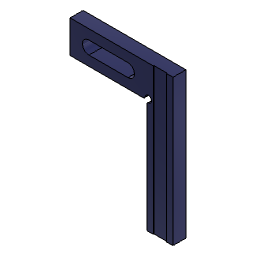
Square_Class (Autodesk Fusion 360 archive; units mm, degrees)
design "Square_Bottom"
Autodesk Fusion 360 part; units mm, degrees
sketch "Sketch1" plane through (0, 0, 0) normal (0, 1, 0) x (1, 0, 0)
  line L0 (0, 0) -> (20, 0)
  line L1 (20, 0) -> (20, -112)
  line L2 (20, -112) -> (-59, -112)
  line L3 (-59, -112) -> (-59, -87)
  line L4 (-59, -87) -> (-2.4388, -87)
  line L5 (0, 0) -> (0, -84.5612)
  line L6 (0, -87) -> (1.0607, -88.0607) construction
  line L7 (0, -87) -> (2, -87) construction
  arc A0 (-1.439, -88.0173) -> (1.0173, -85.561) centre (1.0607, -88.0607) ccw
  arc A1 (0, -84.5612) -> (1.0173, -85.561) centre (1, -84.5612) ccw
  arc A2 (-1.439, -88.0173) -> (-2.4388, -87) centre (-2.4388, -88) ccw
  line L8 (-59, -99.5) -> (-49.5, -99.5) construction
  line L9 (-27.9553, -112) -> (-27.9553, -104.5) construction
  line L10 (-27.9553, -87) -> (-27.9553, -94.5) construction
  line L11 (-14.5, -94.5) -> (-44.5, -94.5)
  line L12 (-44.5, -104.5) -> (-14.5, -104.5)
  arc A3 (-14.5, -104.5) -> (-14.5, -94.5) centre (-14.5, -99.5) ccw
  arc A4 (-44.5, -94.5) -> (-44.5, -104.5) centre (-44.5, -99.5) ccw
  point P0 (0, -85.7968)
  dimension "d1" = 20
  dimension "d2" = 112
  dimension "d3" = 79
  dimension "d5" = 59
  dimension "d8" = 45
  dimension "d9" = 1.5
  dimension "d10" = 5
  dimension "d11" = 25
  dimension "d12" = 85.7968
  dimension "d13" = 1
  dimension "d14" = 9.5
  dimension "d15" = 7.5
  dimension "d16" = 7.5
  dimension "d17" = 10
  dimension "d18" = 30
  dimension "d19" = 10
  constraint coincident L0.start L5.start
  constraint horizontal L0
  constraint perpendicular L0 L1
  constraint perpendicular L1 L2
  constraint perpendicular L2 L3
  constraint perpendicular L3 L4
  constraint horizontal L7
  constraint coincident L6.end A0.centre
  constraint coincident L5 P0
  constraint coincident P0 A0
  constraint tangent L5 A1
  constraint tangent A0 A1
  constraint tangent L4 A2
  constraint tangent A0 A2
  constraint equal A1 A2
  constraint midpoint L3 L8.start
  constraint perpendicular L3 L8
  constraint coincident L2 L9.start
  constraint perpendicular L2 L9
  constraint coincident L4 L10.start
  constraint perpendicular L4 L10
  constraint coincident L8.end A4
  constraint tangent L11 A4
  constraint perpendicular L10 L11
  constraint tangent L12 A3
  constraint perpendicular L9 L12
  measures "d1" distance of L0.start L0.end
  measures "d2" distance of L0.end L1.end
  measures "d3" distance of L1.end L2.end
  measures "d5" distance of L3.end L6.start
  measures "d8" angle of L6 L7
  measures "d9" distance of L6.start L6.end
  measures "d10" diameter of A0
  measures "d11" distance of L2 L4
  measures "d12" distance of L0.start P0
  measures "d13" radius of A1
  measures "d14" distance of L8.start L8.end
  measures "d15" distance of L9.start L9.end
  measures "d16" distance of L10.start L10.end
  measures "d17" diameter of A4
  measures "d18" distance of A4.centre A3.centre
  measures "d19" diameter of A3
extrude "Extrude1" add sketch "Sketch1" along normal blind 10
sketch "Sketch3" plane through (0, 0, 0) normal (0, 1, 0) x (1, 0, 0)
  line L0 (0, 0) -> (5, 0) construction
  line L1 (5, 0) -> (15, 0)
  line L2 (15, 0) -> (15, -120)
  line L3 (15, -120) -> (5, -120)
  line L4 (5, -120) -> (5, 0)
  dimension "d26" = 5
  dimension "d27" = 10
  dimension "d28" = 120
  constraint coincident L0.start origin
  constraint horizontal L0
  constraint horizontal L1
  constraint vertical L2
  constraint horizontal L3
  constraint vertical L4
  measures "d26" distance of L0.start L0.end
  measures "d27" distance of L0.end L1.end
  measures "d28" distance of L0.end L3.end
extrude "Extrude2" cut sketch "Sketch3" along normal blind 0.5
